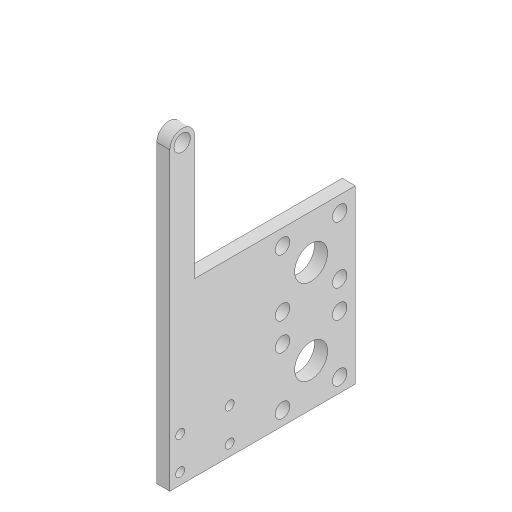
# Autodesk Inventor part: VertialIntakeSlides
Saved by Autodesk Inventor 2023 (Build 270158000, 158)
## iProperties
Created: 2022-11-08
Part Number: VertialIntakeSlides
Material: Generic
Document SubType Name: Modeling
Designer: deli
Density: 1 g/cm^3
Appearance: Default
Author: deli
Autodesk Inventor part; units mm, degrees
ref_plane "YZ Plane" through (0, 0, 0) normal (1, 0, 0) x (0, 1, 0)
ref_plane "XZ Plane" through (0, 0, 0) normal (0, 1, 0) x (-1, 0, 0)
ref_plane "XY Plane" through (0, 0, 0) normal (0, 0, 1) x (1, 0, 0)
sketch "Sketch1" plane through (0, 0, 0) normal (1, 0, 0) x (0, 1, 0)
  line L0 (-55.636, -177.306) -> (-97.1898, -177.306)
  line L1 (-97.1898, -177.306) -> (-97.1898, -222.2006)
  line L2 (-55.636, -222.2006) -> (-97.1898, -222.2006)
  circle A0 centre (-86.4398, -179.806) radius 1.1
  circle A1 centre (-86.4398, -191.806) radius 1.1
  circle A2 centre (-94.4398, -179.806) radius 1.1
  circle A3 centre (-94.4398, -191.806) radius 1.1
  line L3 (-86.4398, -179.806) -> (-94.4398, -179.806) construction
  line L4 (-94.4398, -179.806) -> (-94.4398, -191.806) construction
  line L5 (-94.4398, -191.806) -> (-86.4398, -191.806) construction
  line L6 (-86.4398, -191.806) -> (-86.4398, -179.806) construction
  circle A4 centre (-86.9028, -211.5078) radius 4
  circle A5 centre (-79.988, -204.593) radius 1.778
  circle A6 centre (-79.988, -218.4226) radius 1.778
  circle A7 centre (-93.8176, -218.4226) radius 1.778
  circle A8 centre (-93.8176, -204.593) radius 1.778
  line L7 (-79.988, -204.593) -> (-93.8176, -218.4226) construction
  line L8 (-79.988, -218.4226) -> (-93.8176, -204.593) construction
  line L9 (-93.8176, -204.593) -> (-93.8176, -218.4226) construction
  line L10 (-79.988, -204.593) -> (-79.988, -218.4226) construction
  circle A9 centre (-73.2436, -204.593) radius 1.778
  line L11 (-73.2436, -204.593) -> (-73.2436, -218.4226) construction
  circle A10 centre (-59.414, -204.593) radius 1.778
  circle A11 centre (-73.2436, -218.4226) radius 1.778
  circle A12 centre (-66.3288, -211.5078) radius 4
  line L12 (-59.414, -204.593) -> (-73.2436, -218.4226) construction
  line L13 (-59.414, -218.4226) -> (-73.2436, -204.593) construction
  line L14 (-59.414, -204.593) -> (-59.414, -218.4226) construction
  circle A13 centre (-59.414, -218.4226) radius 1.778
  line L15 (-66.3288, -211.5078) -> (-86.9028, -211.5078) construction
  line L16 (-55.636, -183.306) -> (-55.636, -222.2006)
  line L17 (-55.636, -177.306) -> (-25.636, -177.306)
  line L18 (-25.636, -183.306) -> (-55.636, -183.306)
  arc A14 (-25.636, -183.306) -> (-25.636, -177.306) centre (-25.636, -180.306) ccw
  circle A15 centre (-25.636, -180.306) radius 2
  point P0 (0, 0)
  point P1 (-55.636, -222.2006)
  dimension "d4" = 2.2
  dimension "d5" = 12
  dimension "d6" = 8
  dimension "d7" = 2.75
  dimension "d18" = 8
  dimension "d19" = 3.556
  dimension "d20" = 19.558
  dimension "d21" = 45
  dimension "d22" = 8
  dimension "d23" = 3.556
  dimension "d24" = 19.558
  dimension "d25" = 45
  dimension "d26" = 20.574
  dimension "d27" = 13.8296
  dimension "d32" = 2
  dimension "d33" = 3
  dimension "d34" = 4
  dimension "d36" = 2.5
  dimension "d37" = 12.787
  dimension "d38" = 10.287
  dimension "d39" = 2
  dimension "d40" = 30
  constraints: 38 end point, 16 centre point, 9 equal radius, 7 perpendicular, 5 coincident, 5 midpoint, 4 equal length, 4 horizontal, 2 point on circle, 2 tangent, 2 vertical, 1 parallel
  measures "d4" diameter of A0
  measures "d5" distance of L5.end L3.start
  measures "d6" distance of L3.start L3.end
  measures "d7" distance between parallel lines of L1 L4
  measures "d18" diameter of A4
  measures "d19" diameter of A5
  measures "d20" distance of L10.start L9.end
  measures "d21" angle of L9 L8
  measures "d22" diameter of A12
  measures "d23" diameter of A10
  measures "d24" distance of L14.start L11.end
  measures "d25" angle of L11 L13
  measures "d26" distance of A12.centre A4.centre
  measures "d27" distance of L14.start L14.end
  measures "d32" distance edge to line of A13 L16
  measures "d33" radius of A14
  measures "d34" diameter of A15
  measures "d36" distance between parallel lines of L0 L3
  measures "d37" distance from line of L9.start L5
  measures "d38" distance from line of L1 point (-86.903, -211.508)
  measures "d39" distance edge to line of A6 L2
  measures "d40" distance of L18.start L16.start
extrude "Extrusion1" add sketch "Sketch1" along normal blind 3.175
equation "\"d7\" = -0.5 * d6 + 0.5 * d2"
equation "\"d2\" = 13.5"
body "Solid1"
